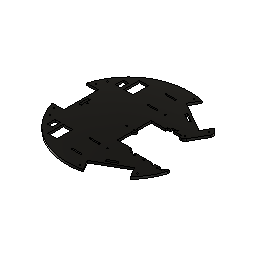
UpperBase v7 (Autodesk Fusion 360 design; units mm, degrees)
Autodesk Fusion 360 part; units mm, degrees
note: some values were not read from the file. Set by a fixed rule: which sketch regions a step uses.
sketch "Sketch1" plane through (0, 0, 0) normal (0, 0, 1) x (1, 0, 0)
  line L0 (-127.0827, 37.5) -> (-102.0827, 37.5)
  line L1 (-102.0827, 37.5) -> (-102.0827, -37.5)
  line L2 (-102.0827, -37.5) -> (-127.0827, -37.5)
  line L3 (0, 0) -> (-132.5, 0) construction
  line L4 (-97.0827, 10) -> (-92.2827, 10)
  line L5 (-92.2827, 10) -> (-92.2827, -10)
  line L6 (-92.2827, -10) -> (-97.0827, -10)
  line L7 (-97.0827, -10) -> (-97.0827, 10)
  arc A0 (-127.0827, 37.5) -> (-132.5, 0) centre (0, 0) ccw construction
  arc A1 (-132.5, 0) -> (-127.0827, -37.5) centre (0, 0) ccw construction
  line L8 (0, 0) -> (66.25, -114.7484) construction
  line L9 (0, 0) -> (66.25, -114.7484) construction
  line L10 (31.0654, -128.8068) -> (18.5654, -107.1562)
  line L11 (18.5654, -107.1562) -> (83.5173, -69.6562)
  line L12 (83.5173, -69.6562) -> (96.0173, -91.3068)
  arc A2 (-127.0827, -37.5) -> (31.0654, -128.8068) centre (0, 0) ccw
  arc A3 (31.0654, -128.8068) -> (66.25, -114.7484) centre (0, 0) ccw construction
  line L13 (37.4811, -84.9191) -> (54.8016, -74.9191)
  line L14 (54.8016, -74.9191) -> (57.2016, -79.076)
  line L15 (57.2016, -79.076) -> (39.8811, -89.076)
  line L16 (39.8811, -89.076) -> (37.4811, -84.9191)
  line L17 (0, 0) -> (132.5, 0) construction
  line L18 (0, 0) -> (66.25, 114.7484) construction
  line L19 (96.0173, 91.3068) -> (83.5173, 69.6562)
  line L20 (83.5173, 69.6562) -> (18.5654, 107.1562)
  line L21 (18.5654, 107.1562) -> (31.0654, 128.8068)
  line L22 (57.2016, 79.076) -> (39.8811, 89.076)
  line L23 (39.8811, 89.076) -> (37.4811, 84.9191)
  line L24 (37.4811, 84.9191) -> (54.8016, 74.9191)
  line L25 (54.8016, 74.9191) -> (57.2016, 79.076)
  circle A4 centre (-115.8879, 45.5) radius 1.5
  circle A5 centre (0, 0) radius 124.5 construction
  circle A6 centre (-115.8879, -45.5) radius 1.5
  circle A7 centre (18.5398, -123.1118) radius 1.5
  circle A8 centre (97.3481, -77.6118) radius 1.5
  circle A9 centre (18.5398, 123.1118) radius 1.5
  arc A10 (66.25, -114.7484) -> (96.0173, -91.3068) centre (0, 0) ccw construction
  arc A11 (96.0173, 91.3068) -> (66.25, 114.7484) centre (0, 0) ccw construction
  arc A12 (31.0654, 128.8068) -> (-127.0827, 37.5) centre (0, 0) ccw
  arc A13 (66.25, 114.7484) -> (31.0654, 128.8068) centre (0, 0) ccw construction
  line L26 (125.8662, 41.4) -> (43.6662, 41.4) construction
  line L27 (43.6662, 41.4) -> (43.6662, -41.4) construction
  line L28 (43.6662, -41.4) -> (125.8662, -41.4) construction
  line L29 (43.6662, 36.6) -> (43.6662, 41.4)
  line L30 (73.6662, 41.4) -> (73.6662, 36.6)
  line L31 (73.6662, 36.6) -> (78.2887, 36.6)
  circle A14 centre (97.3481, 77.6118) radius 1.5
  line L32 (104.2763, 73.6118) -> (85.2169, 40.6)
  circle A15 centre (78.2887, 44.6) radius 1.5
  line L33 (43.6662, -36.6) -> (43.6662, -41.4)
  circle A16 centre (78.2887, -44.6) radius 1.5
  arc A17 (132.5, 0) -> (125.8662, 41.4) centre (0, 0) ccw construction
  arc A18 (103.6034, 82.599) -> (96.0173, 91.3068) centre (0, 0) ccw
  arc A19 (106.9418, 78.2286) -> (103.6034, 82.599) centre (0, 0) ccw construction
  line L34 (106.9418, 78.2286) -> (104.2763, 73.6118) construction
  arc A20 (125.8662, 41.4) -> (106.9418, 78.2286) centre (0, 0) ccw construction
  line L35 (78.2887, 36.6) -> (82.9075, 36.6) construction
  arc A21 (85.2169, 40.6) -> (78.2887, 36.6) centre (78.2887, 44.6) ccw construction
  arc A22 (78.2887, 36.6) -> (85.2169, 40.6) centre (78.2887, 44.6) ccw
  line L36 (85.2169, 40.6) -> (82.9075, 36.6) construction
  line L37 (106.9418, -78.2286) -> (85.6788, -41.4) construction
  arc A23 (125.8662, -41.4) -> (132.5, 0) centre (0, 0) ccw construction
  arc A24 (103.6034, 82.599) -> (104.2763, 73.6118) centre (97.3481, 77.6118) ccw construction
  arc A25 (104.2763, 73.6118) -> (103.6034, 82.599) centre (97.3481, 77.6118) ccw
  arc A26 (96.0173, -91.3068) -> (106.9418, -78.2286) centre (0, 0) ccw
  arc A27 (106.9418, -78.2286) -> (125.8662, -41.4) centre (0, 0) ccw
  line L38 (78.2887, 44.6) -> (78.2887, -44.6) construction
  line L39 (-102.0827, 58.3) -> (9.9173, 58.3) construction
  line L40 (9.9173, 58.3) -> (9.9173, -58.3) construction
  line L41 (9.9173, -58.3) -> (-102.0827, -58.3) construction
  line L42 (-102.0827, -58.3) -> (-102.0827, 58.3) construction
  circle A28 centre (-88.5827, 0) radius 1.5
  circle A29 centre (-3.5827, 0) radius 1.5
  circle A30 centre (-14.5827, -40.8) radius 5 construction
  line L43 (-20.0827, -61.3) -> (-0.0827, -61.3)
  line L44 (-20.0827, -64.3) -> (-0.0827, -64.3)
  arc A31 (-20.0827, -61.3) -> (-20.0827, -64.3) centre (-20.0827, -62.8) ccw
  arc A32 (-0.0827, -64.3) -> (-0.0827, -61.3) centre (-0.0827, -62.8) ccw
  line L45 (-45.0827, -65.3) -> (29.9173, -65.3) construction
  line L46 (29.9173, -65.3) -> (29.9173, -99.3) construction
  line L47 (29.9173, -99.3) -> (-45.0827, -99.3) construction
  line L48 (-45.0827, -99.3) -> (-45.0827, -65.3) construction
  line L49 (-20.0827, -100.3) -> (-0.0827, -100.3)
  line L50 (-20.0827, -103.3) -> (-0.0827, -103.3)
  arc A33 (-20.0827, -100.3) -> (-20.0827, -103.3) centre (-20.0827, -101.8) ccw
  arc A34 (-0.0827, -103.3) -> (-0.0827, -100.3) centre (-0.0827, -101.8) ccw
  line L51 (-20.0827, 61.3) -> (-0.0827, 61.3)
  line L52 (-20.0827, 64.3) -> (-0.0827, 64.3)
  arc A35 (-20.0827, 64.3) -> (-20.0827, 61.3) centre (-20.0827, 62.8) ccw
  arc A36 (-0.0827, 61.3) -> (-0.0827, 64.3) centre (-0.0827, 62.8) ccw
  line L53 (-45.0827, 65.3) -> (29.9173, 65.3) construction
  line L54 (29.9173, 65.3) -> (29.9173, 99.3) construction
  line L55 (29.9173, 99.3) -> (-45.0827, 99.3) construction
  line L56 (-45.0827, 99.3) -> (-45.0827, 65.3) construction
  line L57 (-20.0827, 100.3) -> (-0.0827, 100.3)
  line L58 (-20.0827, 103.3) -> (-0.0827, 103.3)
  arc A37 (-20.0827, 103.3) -> (-20.0827, 100.3) centre (-20.0827, 101.8) ccw
  arc A38 (-0.0827, 100.3) -> (-0.0827, 103.3) centre (-0.0827, 101.8) ccw
  line L59 (125.8662, -41.4) -> (125.8662, -36.6)
  line L60 (125.8662, -36.6) -> (120.8662, -36.6)
  line L61 (120.8662, -36.6) -> (120.8662, -41.4)
  line L62 (43.6662, -41.4) -> (40.4662, -41.4) construction
  line L63 (40.4662, -41.4) -> (40.4662, -36.6) construction
  line L64 (40.4662, -36.6) -> (43.6662, -36.6) construction
  line L65 (43.6662, 41.4) -> (40.4662, 41.4) construction
  line L66 (40.4662, 41.4) -> (40.4662, 36.6) construction
  line L67 (40.4662, 36.6) -> (43.6662, 36.6) construction
  circle A39 centre (107.8662, -46.4) radius 1.5
  line L68 (110.8662, -41.4) -> (110.8662, -45.4)
  line L69 (110.8662, -45.4) -> (116.8662, -45.4)
  line L70 (116.8662, -45.4) -> (116.8662, -41.4)
  line L71 (98.8662, -41.4) -> (98.8662, -45.4)
  line L72 (92.8662, -41.4) -> (92.8662, -45.4)
  line L73 (92.8662, -45.4) -> (98.8662, -45.4)
  line L74 (50.6662, -41.4) -> (50.6662, -45.4)
  line L75 (50.6662, -45.4) -> (56.6662, -45.4)
  line L76 (56.6662, -45.4) -> (56.6662, -41.4)
  circle A40 centre (60.6662, -46.4) radius 1.5
  line L77 (50.6662, 41.4) -> (50.6662, 45.4)
  line L78 (50.6662, 45.4) -> (56.6662, 45.4)
  line L79 (56.6662, 45.4) -> (56.6662, 41.4)
  circle A41 centre (60.6662, 46.4) radius 1.5
  line L80 (43.6662, -41.4) -> (50.6662, -41.4)
  line L81 (56.6662, -41.4) -> (92.8662, -41.4)
  line L82 (98.8662, -41.4) -> (110.8662, -41.4)
  line L83 (116.8662, -41.4) -> (120.8662, -41.4)
  line L84 (43.6662, 41.4) -> (50.6662, 41.4)
  line L85 (56.6662, 41.4) -> (73.6662, 41.4)
  circle A42 centre (12.9173, 0) radius 1.5
  line L86 (12.9173, 36.6) -> (43.6662, 36.6)
  line L87 (12.9173, -36.6) -> (43.6662, -36.6)
  line L88 (17.4993, -62.8) -> (-107.5007, -62.8) construction
  line L89 (17.4993, 62.8) -> (-107.5007, 62.8) construction
  circle A43 centre (-107.5007, 62.8) radius 1.5
  circle A44 centre (17.4993, 62.8) radius 1.5
  circle A45 centre (17.4993, -62.8) radius 1.5
  circle A46 centre (-107.5007, -62.8) radius 1.5
  line L90 (12.9173, 36.6) -> (12.9173, 5)
  line L91 (12.9173, -5) -> (12.9173, -36.6)
  line L92 (-93.4182, 82.3) -> (-81.9182, 82.3)
  line L93 (-81.9182, 82.3) -> (-81.9182, 65.3)
  line L94 (-81.9182, 65.3) -> (-93.4182, 65.3)
  line L95 (-93.4182, 65.3) -> (-93.4182, 82.3)
  line L96 (-93.4182, -82.3) -> (-81.9182, -82.3)
  line L97 (-81.9182, -82.3) -> (-81.9182, -65.3)
  line L98 (-81.9182, -65.3) -> (-93.4182, -65.3)
  line L99 (-93.4182, -65.3) -> (-93.4182, -82.3)
  line L100 (-75.0983, -99.3) -> (-55.0983, -99.3)
  line L101 (-55.0983, -99.3) -> (-55.0983, -65.3)
  line L102 (-75.0983, -65.3) -> (-75.0983, -99.3)
  line L103 (-75.0983, 99.3) -> (-55.0983, 99.3)
  line L104 (-55.0983, 99.3) -> (-55.0983, 65.3)
  line L105 (-55.0983, 65.3) -> (-75.0983, 65.3)
  line L106 (-75.0983, 65.3) -> (-75.0983, 99.3)
  line L107 (-75.0983, -65.3) -> (-55.0983, -65.3)
  line L108 (17.4993, 62.8) -> (17.4993, -62.8) construction
  line L109 (12.9173, 5) -> (12.9173, -5) construction
  arc A47 (12.9173, 5) -> (9.9173, 4) centre (12.9173, 0) ccw construction
  arc A48 (9.9173, 4) -> (9.9173, -4) centre (12.9173, 0) ccw construction
  arc A49 (12.9173, -5) -> (12.9173, 5) centre (12.9173, 0) ccw
  arc A50 (9.9173, -4) -> (12.9173, -5) centre (12.9173, 0) ccw construction
  line L110 (-81.9182, -65.3) -> (-75.0983, -65.3) construction
  line L111 (-81.9182, 65.3) -> (-75.0983, 65.3) construction
  point P0 (-102.0827, 0)
  point P1 (-97.0827, 0)
  point P2 (51.0413, -88.4062)
  point P3 (48.5413, -84.076)
  point P4 (51.0413, 88.4062)
  point P5 (48.5413, 84.076)
  point P6 (43.6662, 0)
  point P7 (78.2887, 0)
  point P8 (-102.0827, 0)
  point P9 (53.6662, 45.4)
  point P10 (53.6662, -45.4)
  point P11 (95.8662, -45.4)
  point P12 (113.8662, -45.4)
  point P13 (12.9173, 0)
  point P14 (17.4993, 0)
  dimension "d1" = 265
  dimension "d2" = 75
  dimension "d3" = 25
  dimension "d4" = 4.8
  dimension "d5" = 20
  dimension "d6" = 5
  dimension "d17" = 120
  dimension "d19" = 132.5
  dimension "d20" = 75
  dimension "d21" = 25
  dimension "d22" = 20
  dimension "d23" = 4.8
  dimension "d24" = 5
  dimension "d25" = 132.5
  dimension "d28" = 60
  dimension "d29" = 75
  dimension "d30" = 25
  dimension "d31" = 4.8
  dimension "d32" = 20
  dimension "d33" = 5
  dimension "d34" = 3
  dimension "d35" = 8
  dimension "d36" = 249
  dimension "d37" = 3
  dimension "d38" = 8
  dimension "d39" = 3
  dimension "d40" = 8
  dimension "d41" = 3
  dimension "d42" = 8
  dimension "d49" = 3
  dimension "d50" = 8
  dimension "d156" = 82.8
  dimension "d157" = 82.2
  dimension "d167" = 3
  dimension "d168" = 8
  dimension "d169" = 8
  dimension "d170" = 3
  dimension "d171" = 8
  dimension "d172" = 8
  dimension "d181" = 3
  dimension "d184" = 8
  dimension "d185" = 8
  dimension "d193" = 116.6
  dimension "d194" = 112
  dimension "d196" = 3
  dimension "d197" = 13.5
  dimension "d198" = 3
  dimension "d199" = 85
  dimension "d200" = 10
  dimension "d201" = 24.5
  dimension "d202" = 17.5
  dimension "d203" = 20
  dimension "d204" = 3
  dimension "d206" = 1
  dimension "d207" = 7
  dimension "d208" = 34
  dimension "d209" = 75
  dimension "d210" = 3
  dimension "d211" = 20
  dimension "d212" = 30
  dimension "d213" = 1
  dimension "d217" = 20
  dimension "d218" = 3
  dimension "d219" = 1
  dimension "d220" = 7
  dimension "d221" = 75
  dimension "d222" = 34
  dimension "d224" = 20
  dimension "d225" = 3
  dimension "d226" = 1
  dimension "d227" = 30
  dimension "d233" = 30
  dimension "d234" = 4.8
  dimension "d238" = 3.2
  dimension "d239" = 4.8
  dimension "d240" = 5
  dimension "d241" = 3.2
  dimension "d242" = 4.8
  dimension "d243" = 3.2
  dimension "d244" = 4.8
  dimension "d245" = 3
  dimension "d246" = 13
  dimension "d247" = 5
  dimension "d248" = 4
  dimension "d249" = 6
  dimension "d250" = 4
  dimension "d252" = 6
  dimension "d253" = 4
  dimension "d254" = 6
  dimension "d255" = 3
  dimension "d256" = 5
  dimension "d257" = 4
  dimension "d258" = 6
  dimension "d259" = 3
  dimension "d260" = 5
  dimension "d261" = 10
  dimension "d262" = 17
  dimension "d263" = 10
  dimension "d264" = 17
  dimension "d266" = 25
  dimension "d267" = 18
  dimension "d269" = 3
  dimension "d274" = 125
  dimension "d276" = 125
  dimension "d277" = 3
  dimension "d278" = 3
  dimension "d279" = 3
  dimension "d280" = 3
  dimension "d286" = 30
  dimension "d287" = 20
  dimension "d288" = 30
  dimension "d290" = 20
  dimension "d291" = 11.5
  dimension "d292" = 17
  dimension "d294" = 7
  dimension "d297" = 11.5
  dimension "d298" = 17
  dimension "d299" = 7
  dimension "d300" = 20
  dimension "d302" = 20
  dimension "d304" = 34
  dimension "d306" = 34
  dimension "d307" = 125.6
  dimension "d308" = 115
  dimension "d309" = 10
  constraint coincident L3.start A0.centre
  constraint horizontal L0
  constraint perpendicular L0 L1
  constraint horizontal L2
  constraint perpendicular L1 L3
  constraint midpoint L1 P0
  constraint coincident L3 P0
  constraint horizontal L4
  constraint vertical L5
  constraint horizontal L6
  constraint vertical L7
  constraint midpoint L7 P1
  constraint coincident L3 P1
  constraint concentric A0 A2
  constraint concentric A1 A2
  constraint coincident L8.end A2
  constraint parallel L8 L10
  constraint perpendicular L8 L11
  constraint coincident L12.end A2
  constraint perpendicular L11 L12
  constraint midpoint L11 P2
  constraint coincident L8 P2
  constraint concentric A2 A3
  constraint perpendicular L12 L13
  constraint perpendicular L13 L14
  constraint perpendicular L9 L15
  constraint parallel L8 L16
  constraint midpoint L15 P3
  constraint coincident L8 P3
  constraint horizontal L17
  constraint parallel L18 L19
  constraint perpendicular L18 L20
  constraint perpendicular L20 L21
  constraint midpoint L20 P4
  constraint coincident L18 P4
  constraint perpendicular L18 L22
  constraint perpendicular L22 L23
  constraint perpendicular L18 L24
  constraint parallel L18 L25
  constraint midpoint L22 P5
  constraint coincident L18 P5
  constraint coincident A4.centre A5
  constraint coincident A5 A6.centre
  constraint coincident A5 A7.centre
  constraint coincident A5 A8.centre
  constraint coincident A5 A9.centre
  constraint coincident L17.end A10
  constraint concentric A10 A11
  constraint concentric A10 A23
  constraint concentric A11 A17
  constraint concentric A11 A12
  constraint concentric A11 A13
  constraint horizontal L26
  constraint perpendicular L26 L27
  constraint perpendicular L27 L28
  constraint midpoint L27 P6
  constraint coincident L17 P6
  constraint perpendicular L30 L31
  constraint coincident A5 A14.centre
  constraint parallel L18 L32
  constraint concentric A15 A21
  constraint tangent L31 A21
  constraint concentric A14 A24
  constraint tangent L32 A24
  constraint concentric A17 A18
  constraint concentric A17 A19
  constraint tangent L34 A24
  constraint concentric A17 A20
  constraint tangent L35 A21
  constraint concentric A21 A22
  constraint tangent L36 A24
  constraint concentric A24 A25
  constraint concentric A23 A26
  constraint concentric A23 A27
  constraint coincident A15.centre A21.centre
  constraint coincident A16.centre L38.end
  constraint perpendicular L28 L38
  constraint midpoint L38 P7
  constraint coincident L17 P7
  constraint horizontal L39
  constraint vertical L40
  constraint horizontal L41
  constraint vertical L42
  constraint midpoint L42 P8
  constraint coincident L3 P8
  constraint coincident L3 A28.centre
  constraint coincident L3 A29.centre
  constraint perpendicular L40 L43
  constraint parallel L43 L44
  constraint tangent L44 A31
  constraint tangent L43 A31
  constraint tangent L43 A32
  constraint tangent L44 A32
  constraint horizontal L45
  constraint vertical L46
  constraint horizontal L47
  constraint vertical L48
  constraint horizontal L49
  constraint parallel L49 L50
  constraint tangent L49 A33
  constraint tangent L50 A33
  constraint tangent L49 A34
  constraint tangent L50 A34
  constraint parallel L39 L51
  constraint parallel L51 L52
  constraint tangent L52 A35
  constraint tangent L51 A35
  constraint tangent L52 A36
  constraint tangent L51 A36
  constraint horizontal L53
  constraint vertical L54
  constraint horizontal L55
  constraint vertical L56
  constraint horizontal L57
  constraint parallel L57 L58
  constraint tangent L58 A37
  constraint tangent L57 A37
  constraint tangent L58 A38
  constraint tangent L57 A38
  constraint coincident L28 L37.end
  constraint tangent A22 L36
  constraint perpendicular L28 L59
  constraint perpendicular L59 L60
  constraint coincident L28 L61.end
  constraint perpendicular L28 L61
  constraint perpendicular L27 L62
  constraint perpendicular L62 L63
  constraint coincident L27 L33.start
  constraint perpendicular L33 L64
  constraint perpendicular L27 L65
  constraint perpendicular L65 L66
  constraint coincident L27 L29.start
  constraint perpendicular L29 L67
  constraint perpendicular L28 L68
  constraint perpendicular L68 L69
  constraint perpendicular L28 L71
  constraint coincident L28 L72.start
  constraint perpendicular L28 L72
  constraint perpendicular L74 L75
  constraint coincident L28 L76.end
  constraint perpendicular L28 L76
  constraint perpendicular L77 L84
  constraint perpendicular L77 L78
  constraint coincident L26 L79.end
  constraint perpendicular L79 L84
  constraint midpoint L78 P9
  constraint midpoint L75 P10
  constraint midpoint L73 P11
  constraint midpoint L69 P12
  constraint perpendicular L74 L80
  constraint perpendicular L68 L82
  constraint perpendicular L61 L83
  constraint perpendicular L33 L80
  constraint perpendicular L70 L83
  constraint perpendicular L79 L85
  constraint coincident L17 P13
  constraint coincident P13 A42.centre
  constraint perpendicular L27 L86
  constraint perpendicular L27 L87
  constraint coincident L89.end A43.centre
  constraint coincident L89.start A44.centre
  constraint coincident L88.start A45.centre
  constraint coincident L88.end A46.centre
  constraint perpendicular L86 L90
  constraint perpendicular L87 L91
  constraint collinear L1 L42
  constraint horizontal L92
  constraint vertical L93
  constraint horizontal L94
  constraint vertical L95
  constraint coincident A5 L92.start
  constraint horizontal L96
  constraint vertical L97
  constraint horizontal L98
  constraint vertical L99
  constraint coincident A5 L96.start
  constraint horizontal L100
  constraint vertical L101
  constraint vertical L102
  constraint coincident A5 L100.start
  constraint horizontal L103
  constraint vertical L104
  constraint horizontal L105
  constraint vertical L106
  constraint coincident A5 L103.start
  constraint perpendicular L101 L107
  constraint perpendicular L88 L108
  constraint coincident A5 L88.end
  constraint horizontal L88
  constraint coincident A5 L89.end
  constraint midpoint L108 P14
  constraint coincident L17 P14
  constraint perpendicular L17 L109
  constraint concentric A42 A48
  constraint coincident L91.start A48
  constraint coincident L40 A47.end
  constraint concentric A47 A48
  constraint coincident L40 A48.end
  constraint concentric A48 A49
  constraint concentric A48 A50
  constraint horizontal L110
  constraint perpendicular L106 L111
  measures "d1" diameter of A2
  measures "d2" distance of L0.end L1.end
  measures "d3" distance of L1.end L2.end
  measures "d4" distance of L4.start L4.end
  measures "d5" distance of L4.end L5.end
  measures "d6" distance of L1 L7
  measures "d17" angle of L3 L8
  measures "d19" distance of L3.start L8.end
  measures "d20" distance of L10.end L11.end
  measures "d21" distance of L10.start L10.end
  measures "d22" distance of L13.start L13.end
  measures "d23" distance of L13.start L15.end
  measures "d24" distance of L11 L15
  measures "d25" distance of L3.start L17.end
  measures "d28" angle of L17 L18
  measures "d29" distance of L19.end L20.end
  measures "d30" distance of L19.start L19.end
  measures "d31" distance of L22.start L24.end
  measures "d32" distance of L23.end L24.end
  measures "d33" distance of L20 L22
  measures "d34" diameter of A4
  measures "d35" distance of L0 A4.centre
  measures "d36" diameter of A5
  measures "d37" diameter of A6
  measures "d38" distance of L2 A6.centre
  measures "d39" diameter of A7
  measures "d40" distance of L10 A7.centre
  measures "d41" diameter of A8
  measures "d42" distance of L12 A8.centre
  measures "d49" diameter of A9
  measures "d50" distance of L21 A9.centre
  measures "d156" distance of L26.end L27.end
  measures "d157" distance of L26.start L26.end
  measures "d167" diameter of A14
  measures "d168" distance of L19 A14.centre
  measures "d169" distance of A14.centre L32
  measures "d170" diameter of A15
  measures "d171" distance of L32 A15.centre
  measures "d172" distance of L31 A15.centre
  measures "d181" diameter of A16
  measures "d184" distance of A16.centre L37
  measures "d185" distance of A8.centre L37
  measures "d193" distance of L39.start L41.end
  measures "d194" distance of L39.start L39.end
  measures "d196" diameter of A28
  measures "d197" distance of L42 A28.centre
  measures "d198" diameter of A29
  measures "d199" distance of A28.centre A29.centre
  measures "d200" diameter of A30
  measures "d201" distance of L40 A30.centre
  measures "d202" distance of L41 A30.centre
  measures "d203" distance of L43.start L43.end
  measures "d204" distance of L43 L44
  measures "d206" distance of L44 L45
  measures "d207" distance of L41 L45
  measures "d208" distance of L45.start L47.end
  measures "d209" distance of L46.end L47.end
  measures "d210" distance of L49 L50
  measures "d211" distance of L50.start L50.end
  measures "d212" distance of L46 A34.centre
  measures "d213" distance of L47 L49
  measures "d217" distance of L51.start L51.end
  measures "d218" distance of L51 L52
  measures "d219" distance of L52 L53
  measures "d220" distance of L39 L53
  measures "d221" distance of L53.start L53.end
  measures "d222" distance of L53.end L54.end
  measures "d224" distance of L58.start L58.end
  measures "d225" distance of L57 L58
  measures "d226" distance of L55 L57
  measures "d227" distance of L54 A38.centre
  measures "d233" distance of L29 L30
  measures "d234" distance of L30.start L30.end
  measures "d238" distance of L28 A16.centre
  measures "d239" distance of L28.end L59.end
  measures "d240" distance of L59.end L60.end
  measures "d241" distance of L27.end L62.end
  measures "d242" distance of L62.end L63.end
  measures "d243" distance of L26.end L65.end
  measures "d244" distance of L65.end L66.end
  measures "d245" diameter of A39
  measures "d246" distance of L61 A39.centre
  measures "d247" distance of L28 A39.centre
  measures "d248" distance of L68.start L68.end
  measures "d249" distance of L68.end L69.end
  measures "d250" distance of L71.start L71.end
  measures "d252" distance of L71.end L72.end
  measures "d253" distance of L74.start L74.end
  measures "d254" distance of L74.end L75.end
  measures "d255" diameter of A40
  measures "d256" distance of L28 A40.centre
  measures "d257" distance of L77.start L77.end
  measures "d258" distance of L77.end L78.end
  measures "d259" diameter of A41
  measures "d260" distance of L26 A41.centre
  measures "d261" horizontal distance of L26.end P9
  measures "d262" horizontal distance of L26.end A41.centre
  measures "d263" horizontal distance of L27.end P10
  measures "d264" horizontal distance of L27.end A40.centre
  measures "d266" horizontal distance of L61.end P11
  measures "d267" distance of P11 P12
  measures "d269" diameter of A42
  measures "d274" distance of L88.start L88.end
  measures "d276" distance of L89.start L89.end
  measures "d277" diameter of A43
  measures "d278" diameter of A44
  measures "d279" diameter of A45
  measures "d280" diameter of A46
  measures "d286" distance of A32.centre L46
  measures "d287" distance of L40 L46
  measures "d288" distance of A36.centre L54
  measures "d290" distance of L40 L54
  measures "d291" distance of L92.start L92.end
  measures "d292" distance of L92.start L94.end
  measures "d294" distance of L39 L94
  measures "d297" distance of L96.start L96.end
  measures "d298" distance of L96.start L98.end
  measures "d299" distance of L41 L98
  measures "d300" distance of L100.start L100.end
  measures "d302" distance of L103.start L103.end
  measures "d304" distance of L103.start L105.end
  measures "d306" distance of L100.end L101.end
  measures "d307" distance of L89.start L88.start
  measures "d308" distance of L42 L90
  measures "d309" diameter of A48
extrude "Extrude1" add sketch "Sketch1" against normal blind 4.8
